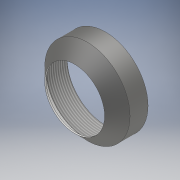
# Autodesk Inventor part: Part 1 of Focusrite Microphone
Saved by Autodesk Inventor 2018 (Build 220112000, 112)
## iProperties
Created: 2017-11-13
Part Number: Part 1 of Focusrite Microphone
Material: Generic
Document SubType Name: Modeling
Designer: Justin
Density: 1 g/cm^3
Appearance: Default
Author: Justin
Autodesk Inventor part; units mm, degrees
ref_plane "YZ Plane" through (0, 0, 0) normal (1, 0, 0) x (0, 1, 0)
ref_plane "XZ Plane" through (0, 0, 0) normal (0, 1, 0) x (-1, 0, 0)
ref_plane "XY Plane" through (0, 0, 0) normal (0, 0, 1) x (1, 0, 0)
sketch "Sketch1" plane through (0, 0, 0) normal (0, 0, 1) x (1, 0, 0)
  line L0 (20, 0) -> (28.4853, 8.4853)
  line L1 (28.4853, 8.4853) -> (28.4853, 20.4853)
  line L2 (28.4853, 20.4853) -> (25.4853, 20.4853)
  line L3 (25.4853, 20.4853) -> (25.4853, 6.4853)
  line L4 (25.4853, 6.4853) -> (20, 1)
  line L5 (20, 1) -> (20, 0)
  line L6 (20, 0) -> (0, 0)
  line L7 (0, 0) -> (0, 1)
  line L8 (0, 1) -> (20, 1)
  dimension "d0" = 20
  dimension "d1" = 12
  dimension "d3" = 12
  dimension "d4" = 3
  dimension "d5" = 14
  constraints: 18 end point, 2 horizontal, 2 parallel, 2 vertical, 1 perpendicular
  measures "d0" distance of L6.end L0.start
  measures "d1" distance of L0.start L0.end
  measures "d3" distance of L0.end L1.end
  measures "d4" distance of L1.end L2.end
  measures "d5" distance of L2.end L3.end
revolve "Revolution1" add sketch "Sketch1" angle 360 about axis through (0, 0, 0) along (0, 1, 0)
thread "Thread1" size "M52x1.5" class "6H" standard "ANSI Metric M Profile" full length
sketch "Sketch2" plane through (0, 0, 0) normal (0, -1, 0) x (1, 0, 0)
  point P0 (0, 0)
hole "Hole1" at (0, 0, 0) direction (0, 1, 0) diameter 40 end through all
body "Solid1"
